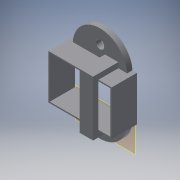
# Autodesk Inventor part: RS485_cover
Saved by Autodesk Inventor 2019.3 (Build 233278000, 278)
## iProperties
Created: 2020-09-10
Part Number: RS485_cover
Material: Generisch
Document SubType Name: Modeling
Designer: Nicolas Frick
Density: 1 g/cm^3
Appearance: Vorgabe
Author: Nicolas Frick
Autodesk Inventor part; units mm, degrees
ref_plane "YZ Plane" through (0, 0, 0) normal (1, 0, 0) x (0, 1, 0)
ref_plane "XZ Plane" through (0, 0, 0) normal (0, 1, 0) x (-1, 0, 0)
ref_plane "XY Plane" through (0, 0, 0) normal (0, 0, 1) x (1, 0, 0)
sketch "Skizze1" plane through (0, 0, 0) normal (0, 0, 1) x (1, 0, 0)
  arc A0 (10.25, -7.75) -> (11.25, -6.75) centre (10.25, -6.75) ccw construction
  line L0 (11.25, -6.75) -> (11.25, 6.75) construction
  arc A1 (11.25, 6.75) -> (10.25, 7.75) centre (10.25, 6.75) ccw construction
  line L1 (10.25, 7.75) -> (-10.25, 7.75) construction
  arc A2 (-10.25, 7.75) -> (-11.25, 6.75) centre (-10.25, 6.75) ccw construction
  line L2 (-11.25, 6.75) -> (-11.25, -6.75) construction
  arc A3 (-11.25, -6.75) -> (-10.25, -7.75) centre (-10.25, -6.75) ccw construction
  line L3 (-10.25, -7.75) -> (10.25, -7.75) construction
  line L4 (10.25, 6.75) -> (10.25, -6.75) construction
  line L5 (10.25, -6.75) -> (-10.25, -6.75) construction
  line L6 (-10.25, -6.75) -> (-10.25, 6.75) construction
  line L7 (-10.25, 6.75) -> (10.25, 6.75) construction
  arc A4 (-10.25, -7.75) -> (10.25, -7.75) centre (0, -7.75) ccw construction
  arc A5 (10.25, 7.75) -> (-10.25, 7.75) centre (0, 7.75) ccw construction
  line L8 (11.4, 7.9) -> (-11.4, 7.9)
  line L9 (-11.4, 7.9) -> (-11.4, -7.9)
  line L10 (-11.4, -7.9) -> (11.4, -7.9)
  line L11 (11.4, -7.9) -> (11.4, 7.9)
  line L12 (11.4, 7.9) -> (-11.4, -7.9) construction
  line L13 (-11.4, 7.9) -> (11.4, -7.9) construction
  line L14 (11.9, 8.4) -> (-11.9, 8.4)
  line L15 (-11.9, 8.4) -> (-11.9, -8.4)
  line L16 (-11.9, -8.4) -> (11.9, -8.4)
  line L17 (11.9, -8.4) -> (11.9, 8.4)
  line L18 (11.9, 8.4) -> (-11.9, -8.4) construction
  line L19 (-11.9, 8.4) -> (11.9, -8.4) construction
  point P0 (0, 0)
  dimension "d0" = 22.8
  dimension "d1" = 15.8
  dimension "d2" = 23.8
  dimension "d3" = 16.8
  constraints: 24 end point, 4 midpoint, 4 parallel, 2 horizontal, 2 perpendicular
  measures "d0" distance of L10.end L9.end
  measures "d1" distance of L9.end L8.end
  measures "d2" distance of L16.end L15.end
  measures "d3" distance of L15.end L14.end
ref_plane "Arbeitsebene1" through (-10.25, -18, -9.5) normal (0, 0, 1) x (1, 0, 0)
extrude "Extrusion1" add sketch "Skizze1" against normal up to surface (9.5 mm away)
sketch "Skizze2" plane through (0, 0, 0) normal (0, 0, 1) x (1, 0, 0)
  line L0 (11.4, -7.9) -> (11.4, 7.9) construction
  line L1 (-11.4, 7.9) -> (11.4, 7.9) construction
  line L2 (6.9, -7.9) -> (6.9, 7.9)
  line L3 (1.9, -7.9) -> (1.9, 7.9)
  line L4 (11.9, 8.4) -> (-11.9, 8.4) projected
  line L5 (6.9, -8.4019) -> (1.9, -8.4019)
  line L6 (1.9, -8.4019) -> (1.9, 8.4)
  line L7 (1.9, 8.4) -> (6.9, 8.4)
  line L8 (6.9, 8.4) -> (6.9, -8.4019)
  point P0 (0, 0)
  constraints: 12 end point, 3 point on line, 2 parallel, 1 horizontal, 1 perpendicular
extrude "Extrusion2" add sketch "Skizze2" along normal blind 2
sketch "Skizze3" plane through (0, 0, 2) normal (0, 0, 1) x (1, 0, 0)
  line L0 (1.9, -8.4019) -> (6.9, -8.4019) projected
  line L1 (6.9, -8.4019) -> (1.9, -8.4019)
  line L2 (1.9, -8.4019) -> (1.9, -10.4019)
  line L3 (1.9, -10.4019) -> (6.9, -10.4019)
  line L4 (6.9, -10.4019) -> (6.9, -8.4019)
  line L5 (6.9, 8.4) -> (1.9, 8.4) projected
  line L6 (6.9, 8.4) -> (1.9, 8.4)
  line L7 (1.9, 8.4) -> (1.9, 10.4)
  line L8 (1.9, 10.4) -> (6.9, 10.4)
  line L9 (6.9, 10.4) -> (6.9, 8.4)
  point P0 (0, 0)
  dimension "d10" = 2
  dimension "d11" = 2
  constraints: 16 end point, 4 parallel, 2 horizontal, 2 perpendicular, 1 point on line
  measures "d10" distance of L2.end L1.end
  measures "d11" distance of L6.end L7.end
ref_plane "Arbeitsebene2" through (-10.25, -18, -9.5) normal (0, 0, 1) x (1, 0, 0)
extrude "Extrusion3" add sketch "Skizze3" against normal up to surface (11.5 mm away)
ref_plane "Arbeitsebene3" through (0, 0, -9.5) normal (0, 0, 1) x (1, 0, 0)
sketch "Skizze4" plane through (0, 0, -9.5) normal (0, 0, 1) x (1, 0, 0)
  arc A0 (-10.25, -7.75) -> (10.25, -7.75) centre (0, -7.75) ccw projected
  line L0 (-11.9, -8.4) -> (1.9, -8.4) projected
  line L1 (1.9, -10.4019) -> (1.9, 10.4) construction
  line L2 (1.9, -10.4019) -> (6.9, -10.4019) projected
  line L3 (6.9, -10.4019) -> (6.9, 10.4) construction
  line L4 (6.9, -8.4) -> (11.9, -8.4) projected
  line L5 (11.9, 8.4) -> (6.9, 8.4) projected
  line L6 (1.9, 10.4) -> (6.9, 10.4) projected
  line L7 (1.9, 8.4) -> (-11.9, 8.4) projected
  arc A1 (10.25, 7.75) -> (-10.25, 7.75) centre (0, 7.75) ccw projected
  line L8 (1.9, -10.4019) -> (1.9, -8.4)
  line L9 (6.9, -10.4019) -> (6.9, -8.4)
  line L10 (6.9, 10.4) -> (6.9, 8.4) projected
  line L11 (6.9, 10.4) -> (6.9, 8.4)
  line L12 (1.9, 8.4) -> (1.9, 10.4) projected
  line L13 (1.9, 8.4) -> (1.9, 10.4)
  line L14 (10.2294, 8.4) -> (-10.2294, 8.4)
  line L15 (-10.2294, -8.4) -> (10.2294, -8.4)
  line L16 (6.9, -10.4019) -> (1.9, -10.4019)
  line L17 (6.9, 10.4) -> (1.9, 10.4)
  arc A2 (-10.2294, -8.4) -> (10.2294, -8.4) centre (0, -7.75) ccw
  arc A3 (6.9, -0.1703) -> (6.7082, 0) centre (0, -7.75) ccw
  arc A4 (6.7082, 0) -> (6.9, 0.1703) centre (0, 7.75) ccw
  arc A5 (10.2294, 8.4) -> (-10.2294, 8.4) centre (0, 7.75) ccw
  circle A6 centre (0, 12.75) radius 1.6 projected
  circle A7 centre (0, -12.75) radius 1.6 projected
  point P0 (0, 0)
  constraints: 16 end point, 8 point on circle, 6 point on line, 5 collinear, 4 centre point, 2 coincident, 1 vertical
extrude "Extrusion4" add sketch "Skizze4" along normal blind 2 contours L0 L8 L2 L9 L4 A0 | L5 L10 L6 L12 L7 A1 | A6 | A7
sketch "Skizze5" plane through (0, 0, -7.5) normal (0, 0, 1) x (1, 0, 0)
  line L0 (-10.2294, -8.4) -> (1.9, -8.4) construction
  arc A0 (-10.2294, -8.4) -> (10.2294, -8.4) centre (0, -7.75) ccw construction
  line L1 (6.9, -8.4) -> (10.2294, -8.4) construction
  line L2 (6.9, -8.4) -> (6.9, -8.4019) construction
  line L3 (6.9, -10.4019) -> (6.9, -8.4019) construction
  line L4 (1.9, -10.4019) -> (6.9, -10.4019) construction
  line L5 (1.9, -8.4019) -> (1.9, -10.4019) construction
  line L6 (1.9, -8.4019) -> (1.9, -8.4) construction
  circle A1 centre (0, -12.75) radius 1.6 construction
  circle A2 centre (0, 12.75) radius 1.6 projected
  circle A3 centre (0, -12.75) radius 1.6 projected
  point P0 (0, 0)
extrude "Extrusion5" cut sketch "Skizze5" against normal through all
